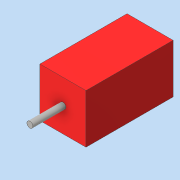
# Autodesk Inventor part: Jinlong_Z4TH5B1241992_VibrationMotor_NoHub_Mockup
Saved by Autodesk Inventor 2016 (Build 200138000, 138)
## iProperties
Created: 2017-10-09
Part Number: Jinlong_Z4TH5B1241992_VibrationMotor_NoHub_Mockup
Material: Generic
Document SubType Name: Modeling
Designer: rahul
Density: 1 g/cm^3
Appearance: Default
Author: rahul
Autodesk Inventor part; units mm, degrees
ref_plane "YZ Plane" through (0, 0, 0) normal (1, 0, 0) x (0, 1, 0)
ref_plane "XZ Plane" through (0, 0, 0) normal (0, 1, 0) x (-1, 0, 0)
ref_plane "XY Plane" through (0, 0, 0) normal (0, 0, 1) x (1, 0, 0)
sketch "Sketch1" plane through (0, 0, 0) normal (0, 0, 1) x (1, 0, 0)
  line L0 (-2.3, 2.45) -> (2.3, 2.45)
  line L1 (2.3, 2.45) -> (2.3, -2.45)
  line L2 (2.3, -2.45) -> (-2.3, -2.45)
  line L3 (-2.3, -2.45) -> (-2.3, 2.45)
  line L4 (0, 3.43) -> (0, -3.43) projected
  line L5 (-3.22, 0) -> (3.22, 0) projected
  point P0 (0, 0)
  dimension "d0" = 4.6
  dimension "d1" = 4.9
  constraints: 8 end point, 2 parallel, 1 horizontal, 1 perpendicular, 2 other
  measures "d0" distance of L0.start L0.end
  measures "d1" distance of L0.end L1.end
extrude "Body" add sketch "Sketch1" against normal blind 8.7
sketch "Sketch2" plane through (0, 0, 0) normal (0, 0, 1) x (1, 0, 0)
  circle A0 centre (0, 0) radius 0.3
  dimension "d4" = 0.6
  constraints: 1 centre point, 1 coincident
  measures "d4" diameter of A0
extrude "Extrusion2" add sketch "Sketch2" along normal blind 3.3
body "Solid1"
